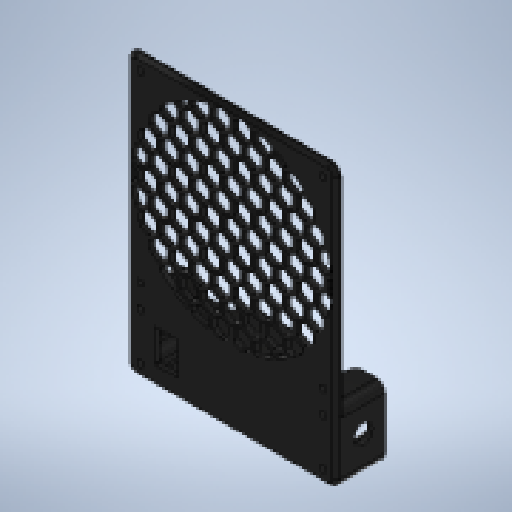
# Autodesk Inventor part: Face Plate
Saved by Autodesk Inventor 2023.2 (Build 272271000, 271)
## iProperties
Created: 2023-08-15
Part Number: Face Plate
Material: UHMW, Black
Document SubType Name: Modeling
Designer: Nathan Cai
Density: 0.94 g/cm^3
Appearance: Smooth - Black
Author: Nathan Cai
Autodesk Inventor part; units mm, degrees
ref_plane "YZ Plane" through (0, 0, 0) normal (1, 0, 0) x (0, 1, 0)
ref_plane "XZ Plane" through (0, 0, 0) normal (0, 1, 0) x (-1, 0, 0)
ref_plane "XY Plane" through (0, 0, 0) normal (0, 0, 1) x (1, 0, 0)
sketch "Sketch1" plane through (0, 0, 0) normal (0, 0, 1) x (1, 0, 0)
  line L0 (-60, -80) -> (60, -80)
  line L1 (60, -80) -> (60, 80)
  line L2 (60, 80) -> (-60, 80)
  line L3 (-60, 80) -> (-60, -80)
  line L4 (-60, -80) -> (60, 80) construction
  line L5 (60, -80) -> (-60, 80) construction
  line L6 (0, 80) -> (0, -80) construction
  line L7 (-52.5, 72.5) -> (52.5, 72.5) construction
  line L8 (52.5, 72.5) -> (52.5, -32.5) construction
  line L9 (52.5, -32.5) -> (-52.5, -32.5) construction
  line L10 (-52.5, -32.5) -> (-52.5, 72.5) construction
  line L11 (-52.5, 72.5) -> (52.5, -32.5) construction
  line L12 (52.5, 72.5) -> (-52.5, -32.5) construction
  circle A0 centre (-52.5, 72.5) radius 2
  circle A1 centre (52.5, 72.5) radius 2
  circle A2 centre (-52.5, -32.5) radius 2
  circle A3 centre (52.5, -32.5) radius 2
  circle A4 centre (-52.5, -72.5) radius 2
  circle A5 centre (52.5, -72.5) radius 2
  circle A6 centre (0, 20) radius 57.5
  circle A7 centre (52.5, -45.5) radius 2
  circle A8 centre (-52.5, -45.5) radius 2
  point P0 (0, 0)
  point P1 (0, 20)
  dimension "d0" = 120
  dimension "d1" = 160
  dimension "d2" = 105
  dimension "d3" = 105
  dimension "d4" = 7.5
  dimension "d5" = 4
  dimension "d8" = 105
  dimension "d11" = 105
  dimension "d16" = 40
  dimension "d21" = 115
  dimension "d82" = 13
  constraints: 26 end point, 9 centre point, 6 midpoint, 4 parallel, 3 horizontal, 3 vertical, 2 coincident, 2 perpendicular, 1 point on line, 14 other
  measures "d0" distance of L2.end L1.end
  measures "d1" distance of L1.end L0.end
  measures "d2" distance of L8.end L9.end
  measures "d3" distance of L7.end L8.end
  measures "d4" distance between parallel lines of L2 L7
  measures "d5" diameter of A0
  measures "d8" distance of A0.centre A1.centre
  measures "d11" distance of A0.centre A2.centre
  measures "d16" distance of A2.centre A4.centre
  measures "d21" diameter of A6
  measures "d82" distance of A3.centre A7.centre
extrude "Extrusion1" add sketch "Sketch1" along normal blind 3
sketch "Sketch2" plane through (0, 0, 3) normal (0, 0, 1) x (1, 0, 0)
  line L0 (60, -80) -> (60, 80) projected
  line L1 (60, 80) -> (-60, 80) projected
  line L2 (-60, 80) -> (-60, -80) projected
  line L3 (-60, -80) -> (60, -80) projected
  circle A0 centre (-52.5, -72.5) radius 2 projected
  circle A1 centre (52.5, -72.5) radius 2 projected
  circle A2 centre (0, 20) radius 57.5 projected
  circle A3 centre (52.5, -32.5) radius 2 projected
  circle A4 centre (-52.5, -32.5) radius 2 projected
  circle A5 centre (52.5, 72.5) radius 2 projected
  circle A6 centre (-52.5, 72.5) radius 2 projected
  circle A7 centre (0, 20) radius 18
  circle A8 centre (0, 20) radius 57.5 projected
  line L4 (0, 77.5) -> (0, -37.5) construction
  line L5 (0, 20) -> (-57.5, 20) construction
  line L6 (0, 25.7735) -> (5, 22.8868)
  line L7 (5, 22.8868) -> (5, 17.1132)
  line L8 (5, 17.1132) -> (0, 14.2265)
  line L9 (0, 14.2265) -> (-5, 17.1132)
  line L10 (-5, 17.1132) -> (-5, 22.8868)
  line L11 (-5, 22.8868) -> (0, 25.7735)
  line L12 (-17, 22.8868) -> (-12, 25.7735)
  line L13 (-7, 17.1132) -> (-12, 14.2265)
  line L14 (-12, 14.2265) -> (-17, 17.1132)
  line L15 (-17, 17.1132) -> (-17, 22.8868)
  line L16 (-7, 22.8868) -> (-7, 17.1132)
  line L17 (-12, 25.7735) -> (-7, 22.8868)
  line L18 (-29, 22.8868) -> (-24, 25.7735)
  line L19 (-19, 17.1132) -> (-24, 14.2265)
  line L20 (-24, 14.2265) -> (-29, 17.1132)
  line L21 (-29, 17.1132) -> (-29, 22.8868)
  line L22 (-19, 22.8868) -> (-19, 17.1132)
  line L23 (-24, 25.7735) -> (-19, 22.8868)
  line L24 (-41, 22.8868) -> (-36, 25.7735)
  line L25 (-31, 17.1132) -> (-36, 14.2265)
  line L26 (-36, 14.2265) -> (-41, 17.1132)
  line L27 (-41, 17.1132) -> (-41, 22.8868)
  line L28 (-31, 22.8868) -> (-31, 17.1132)
  line L29 (-36, 25.7735) -> (-31, 22.8868)
  line L30 (-53, 22.8868) -> (-48, 25.7735)
  line L31 (-43, 17.1132) -> (-48, 14.2265)
  line L32 (-48, 14.2265) -> (-53, 17.1132)
  line L33 (-53, 17.1132) -> (-53, 22.8868)
  line L34 (-43, 22.8868) -> (-43, 17.1132)
  line L35 (-48, 25.7735) -> (-43, 22.8868)
  line L36 (-65, 22.8868) -> (-60, 25.7735)
  line L37 (-55, 17.1132) -> (-60, 14.2265)
  line L38 (-60, 14.2265) -> (-65, 17.1132)
  line L39 (-65, 17.1132) -> (-65, 22.8868)
  line L40 (-55, 22.8868) -> (-55, 17.1132)
  line L41 (-60, 25.7735) -> (-55, 22.8868)
  line L42 (-6, 24.6188) -> (-11, 27.5056)
  line L43 (-11, 27.5056) -> (-11, 33.2791)
  line L44 (-11, 33.2791) -> (-6, 36.1658)
  line L45 (-6, 36.1658) -> (-1, 33.2791)
  line L46 (-1, 33.2791) -> (-1, 27.5056)
  line L47 (-1, 27.5056) -> (-6, 24.6188)
  line L48 (-18, 36.1658) -> (-13, 33.2791)
  line L49 (-13, 33.2791) -> (-13, 27.5056)
  line L50 (-13, 27.5056) -> (-18, 24.6188)
  line L51 (-23, 33.2791) -> (-18, 36.1658)
  line L52 (-23, 27.5056) -> (-23, 33.2791)
  line L53 (-18, 24.6188) -> (-23, 27.5056)
  line L54 (-30, 36.1658) -> (-25, 33.2791)
  line L55 (-25, 33.2791) -> (-25, 27.5056)
  line L56 (-25, 27.5056) -> (-30, 24.6188)
  line L57 (-35, 33.2791) -> (-30, 36.1658)
  line L58 (-35, 27.5056) -> (-35, 33.2791)
  line L59 (-30, 24.6188) -> (-35, 27.5056)
  line L60 (-42, 36.1658) -> (-37, 33.2791)
  line L61 (-37, 33.2791) -> (-37, 27.5056)
  line L62 (-37, 27.5056) -> (-42, 24.6188)
  line L63 (-47, 33.2791) -> (-42, 36.1658)
  line L64 (-47, 27.5056) -> (-47, 33.2791)
  line L65 (-42, 24.6188) -> (-47, 27.5056)
  line L66 (-54, 36.1658) -> (-49, 33.2791)
  line L67 (-49, 33.2791) -> (-49, 27.5056)
  line L68 (-49, 27.5056) -> (-54, 24.6188)
  line L69 (-59, 33.2791) -> (-54, 36.1658)
  line L70 (-59, 27.5056) -> (-59, 33.2791)
  line L71 (-54, 24.6188) -> (-59, 27.5056)
  line L72 (5, 43.6714) -> (5, 37.8979)
  line L73 (-5, 43.6714) -> (0, 46.5581)
  line L74 (-1, 48.2902) -> (-6, 45.4034)
  line L75 (-7, 43.6714) -> (-7, 37.8979)
  line L76 (0, 46.5581) -> (5, 43.6714)
  line L77 (-5, 37.8979) -> (-5, 43.6714)
  line L78 (-12, 46.5581) -> (-7, 43.6714)
  line L79 (-6, 45.4034) -> (-11, 48.2902)
  line L80 (5, 37.8979) -> (0, 35.0111)
  line L81 (0, 35.0111) -> (-5, 37.8979)
  line L82 (-7, 37.8979) -> (-12, 35.0111)
  line L83 (-11, 48.2902) -> (-11, 54.0637)
  line L84 (-1, 54.0637) -> (-1, 48.2902)
  line L85 (-11, 54.0637) -> (-6, 56.9504)
  line L86 (-6, 56.9504) -> (-1, 54.0637)
  line L87 (-24, 35.0111) -> (-29, 37.8979)
  line L88 (-29, 37.8979) -> (-29, 43.6714)
  line L89 (-31, 43.6714) -> (-31, 37.8979)
  line L90 (-31, 37.8979) -> (-36, 35.0111)
  line L91 (-41, 37.8979) -> (-41, 43.6714)
  line L92 (-36, 35.0111) -> (-41, 37.8979)
  line L93 (-53, 37.8979) -> (-53, 43.6714)
  line L94 (-48, 35.0111) -> (-53, 37.8979)
  line L95 (-43, 37.8979) -> (-48, 35.0111)
  line L96 (-43, 43.6714) -> (-43, 37.8979)
  line L97 (-65, 43.6714) -> (-60, 46.5581)
  line L98 (-60, 46.5581) -> (-55, 43.6714)
  line L99 (-55, 43.6714) -> (-55, 37.8979)
  line L100 (-55, 37.8979) -> (-60, 35.0111)
  line L101 (-65, 37.8979) -> (-65, 43.6714)
  line L102 (-60, 35.0111) -> (-65, 37.8979)
  line L103 (-17, 43.6714) -> (-12, 46.5581)
  line L104 (-12, 35.0111) -> (-17, 37.8979)
  line L105 (-17, 37.8979) -> (-17, 43.6714)
  line L106 (-19, 37.8979) -> (-24, 35.0111)
  line L107 (-13, 54.0637) -> (-13, 48.2902)
  line L108 (-18, 56.9504) -> (-13, 54.0637)
  line L109 (-13, 48.2902) -> (-18, 45.4034)
  line L110 (-23, 54.0637) -> (-18, 56.9504)
  line L111 (-23, 48.2902) -> (-23, 54.0637)
  line L112 (-18, 45.4034) -> (-23, 48.2902)
  line L113 (-19, 43.6714) -> (-19, 37.8979)
  line L114 (-24, 46.5581) -> (-19, 43.6714)
  line L115 (-29, 43.6714) -> (-24, 46.5581)
  line L116 (-36, 46.5581) -> (-31, 43.6714)
  line L117 (-41, 43.6714) -> (-36, 46.5581)
  line L118 (-30, 45.4034) -> (-35, 48.2902)
  line L119 (-37, 48.2902) -> (-42, 45.4034)
  line L120 (-25, 48.2902) -> (-30, 45.4034)
  line L121 (-42, 56.9504) -> (-37, 54.0637)
  line L122 (-37, 54.0637) -> (-37, 48.2902)
  line L123 (-35, 54.0637) -> (-30, 56.9504)
  line L124 (-25, 54.0637) -> (-25, 48.2902)
  line L125 (-30, 56.9504) -> (-25, 54.0637)
  line L126 (-35, 48.2902) -> (-35, 54.0637)
  line L127 (-53, 43.6714) -> (-48, 46.5581)
  line L128 (-48, 46.5581) -> (-43, 43.6714)
  line L129 (-42, 45.4034) -> (-47, 48.2902)
  line L130 (-49, 48.2902) -> (-54, 45.4034)
  line L131 (-54, 45.4034) -> (-59, 48.2902)
  line L132 (-47, 54.0637) -> (-42, 56.9504)
  line L133 (-49, 54.0637) -> (-49, 48.2902)
  line L134 (-54, 56.9504) -> (-49, 54.0637)
  line L135 (-59, 48.2902) -> (-59, 54.0637)
  line L136 (-59, 54.0637) -> (-54, 56.9504)
  line L137 (-47, 48.2902) -> (-47, 54.0637)
  line L138 (5, 64.456) -> (5, 58.6825)
  line L139 (-5, 64.456) -> (0, 67.3427)
  line L140 (-1, 69.0748) -> (-6, 66.188)
  line L141 (-7, 64.456) -> (-7, 58.6825)
  line L142 (0, 67.3427) -> (5, 64.456)
  line L143 (-5, 58.6825) -> (-5, 64.456)
  line L144 (-12, 67.3427) -> (-7, 64.456)
  line L145 (-6, 66.188) -> (-11, 69.0748)
  line L146 (5, 58.6825) -> (0, 55.7957)
  line L147 (0, 55.7957) -> (-5, 58.6825)
  line L148 (-7, 58.6825) -> (-12, 55.7957)
  line L149 (-11, 69.0748) -> (-11, 74.8483)
  line L150 (-1, 74.8483) -> (-1, 69.0748)
  line L151 (-11, 74.8483) -> (-6, 77.735)
  line L152 (-6, 77.735) -> (-1, 74.8483)
  line L153 (-24, 55.7957) -> (-29, 58.6825)
  line L154 (-29, 58.6825) -> (-29, 64.456)
  line L155 (-31, 64.456) -> (-31, 58.6825)
  line L156 (-31, 58.6825) -> (-36, 55.7957)
  line L157 (-41, 58.6825) -> (-41, 64.456)
  line L158 (-36, 55.7957) -> (-41, 58.6825)
  line L159 (-53, 58.6825) -> (-53, 64.456)
  line L160 (-48, 55.7957) -> (-53, 58.6825)
  line L161 (-43, 58.6825) -> (-48, 55.7957)
  line L162 (-43, 64.456) -> (-43, 58.6825)
  line L163 (-65, 64.456) -> (-60, 67.3427)
  line L164 (-60, 67.3427) -> (-55, 64.456)
  line L165 (-55, 64.456) -> (-55, 58.6825)
  line L166 (-55, 58.6825) -> (-60, 55.7957)
  line L167 (-65, 58.6825) -> (-65, 64.456)
  line L168 (-60, 55.7957) -> (-65, 58.6825)
  line L169 (-17, 64.456) -> (-12, 67.3427)
  line L170 (-12, 55.7957) -> (-17, 58.6825)
  line L171 (-17, 58.6825) -> (-17, 64.456)
  line L172 (-19, 58.6825) -> (-24, 55.7957)
  line L173 (-13, 74.8483) -> (-13, 69.0748)
  line L174 (-18, 77.735) -> (-13, 74.8483)
  line L175 (-13, 69.0748) -> (-18, 66.188)
  line L176 (-23, 74.8483) -> (-18, 77.735)
  line L177 (-23, 69.0748) -> (-23, 74.8483)
  line L178 (-18, 66.188) -> (-23, 69.0748)
  line L179 (-19, 64.456) -> (-19, 58.6825)
  line L180 (-24, 67.3427) -> (-19, 64.456)
  line L181 (-29, 64.456) -> (-24, 67.3427)
  line L182 (-36, 67.3427) -> (-31, 64.456)
  line L183 (-41, 64.456) -> (-36, 67.3427)
  line L184 (-30, 66.188) -> (-35, 69.0748)
  line L185 (-37, 69.0748) -> (-42, 66.188)
  line L186 (-25, 69.0748) -> (-30, 66.188)
  line L187 (-42, 77.735) -> (-37, 74.8483)
  line L188 (-37, 74.8483) -> (-37, 69.0748)
  line L189 (-35, 74.8483) -> (-30, 77.735)
  line L190 (-25, 74.8483) -> (-25, 69.0748)
  line L191 (-30, 77.735) -> (-25, 74.8483)
  line L192 (-35, 69.0748) -> (-35, 74.8483)
  line L193 (-53, 64.456) -> (-48, 67.3427)
  line L194 (-48, 67.3427) -> (-43, 64.456)
  line L195 (-42, 66.188) -> (-47, 69.0748)
  line L196 (-49, 69.0748) -> (-54, 66.188)
  line L197 (-54, 66.188) -> (-59, 69.0748)
  line L198 (-47, 74.8483) -> (-42, 77.735)
  line L199 (-49, 74.8483) -> (-49, 69.0748)
  line L200 (-54, 77.735) -> (-49, 74.8483)
  line L201 (-59, 69.0748) -> (-59, 74.8483)
  line L202 (-59, 74.8483) -> (-54, 77.735)
  line L203 (-47, 69.0748) -> (-47, 74.8483)
  line L204 (17, 22.8868) -> (12, 25.7735)
  line L205 (7, 17.1132) -> (12, 14.2265)
  line L206 (12, 14.2265) -> (17, 17.1132)
  line L207 (17, 17.1132) -> (17, 22.8868)
  line L208 (7, 22.8868) -> (7, 17.1132)
  line L209 (12, 25.7735) -> (7, 22.8868)
  line L210 (29, 22.8868) -> (24, 25.7735)
  line L211 (19, 17.1132) -> (24, 14.2265)
  line L212 (24, 14.2265) -> (29, 17.1132)
  line L213 (29, 17.1132) -> (29, 22.8868)
  line L214 (19, 22.8868) -> (19, 17.1132)
  line L215 (24, 25.7735) -> (19, 22.8868)
  line L216 (41, 22.8868) -> (36, 25.7735)
  line L217 (31, 17.1132) -> (36, 14.2265)
  line L218 (36, 14.2265) -> (41, 17.1132)
  line L219 (41, 17.1132) -> (41, 22.8868)
  line L220 (31, 22.8868) -> (31, 17.1132)
  line L221 (36, 25.7735) -> (31, 22.8868)
  line L222 (53, 22.8868) -> (48, 25.7735)
  line L223 (43, 17.1132) -> (48, 14.2265)
  line L224 (48, 14.2265) -> (53, 17.1132)
  line L225 (53, 17.1132) -> (53, 22.8868)
  line L226 (43, 22.8868) -> (43, 17.1132)
  line L227 (48, 25.7735) -> (43, 22.8868)
  line L228 (65, 22.8868) -> (60, 25.7735)
  line L229 (55, 17.1132) -> (60, 14.2265)
  line L230 (60, 14.2265) -> (65, 17.1132)
  line L231 (65, 17.1132) -> (65, 22.8868)
  line L232 (55, 22.8868) -> (55, 17.1132)
  line L233 (60, 25.7735) -> (55, 22.8868)
  line L234 (6, 24.6188) -> (11, 27.5056)
  line L235 (11, 27.5056) -> (11, 33.2791)
  line L236 (11, 33.2791) -> (6, 36.1658)
  line L237 (6, 36.1658) -> (1, 33.2791)
  line L238 (1, 33.2791) -> (1, 27.5056)
  line L239 (1, 27.5056) -> (6, 24.6188)
  line L240 (18, 36.1658) -> (13, 33.2791)
  line L241 (13, 33.2791) -> (13, 27.5056)
  line L242 (13, 27.5056) -> (18, 24.6188)
  line L243 (23, 33.2791) -> (18, 36.1658)
  line L244 (23, 27.5056) -> (23, 33.2791)
  line L245 (18, 24.6188) -> (23, 27.5056)
  line L246 (30, 36.1658) -> (25, 33.2791)
  line L247 (25, 33.2791) -> (25, 27.5056)
  line L248 (25, 27.5056) -> (30, 24.6188)
  line L249 (35, 33.2791) -> (30, 36.1658)
  line L250 (35, 27.5056) -> (35, 33.2791)
  line L251 (30, 24.6188) -> (35, 27.5056)
  line L252 (42, 36.1658) -> (37, 33.2791)
  line L253 (37, 33.2791) -> (37, 27.5056)
  line L254 (37, 27.5056) -> (42, 24.6188)
  line L255 (47, 33.2791) -> (42, 36.1658)
  line L256 (47, 27.5056) -> (47, 33.2791)
  line L257 (42, 24.6188) -> (47, 27.5056)
  line L258 (54, 36.1658) -> (49, 33.2791)
  line L259 (49, 33.2791) -> (49, 27.5056)
  line L260 (49, 27.5056) -> (54, 24.6188)
  line L261 (59, 33.2791) -> (54, 36.1658)
  line L262 (59, 27.5056) -> (59, 33.2791)
  line L263 (54, 24.6188) -> (59, 27.5056)
  line L264 (1, 48.2902) -> (6, 45.4034)
  line L265 (7, 43.6714) -> (7, 37.8979)
  line L266 (12, 46.5581) -> (7, 43.6714)
  line L267 (6, 45.4034) -> (11, 48.2902)
  line L268 (7, 37.8979) -> (12, 35.0111)
  line L269 (11, 48.2902) -> (11, 54.0637)
  line L270 (1, 54.0637) -> (1, 48.2902)
  line L271 (11, 54.0637) -> (6, 56.9504)
  line L272 (6, 56.9504) -> (1, 54.0637)
  line L273 (24, 35.0111) -> (29, 37.8979)
  line L274 (29, 37.8979) -> (29, 43.6714)
  line L275 (31, 43.6714) -> (31, 37.8979)
  line L276 (31, 37.8979) -> (36, 35.0111)
  line L277 (41, 37.8979) -> (41, 43.6714)
  line L278 (36, 35.0111) -> (41, 37.8979)
  line L279 (53, 37.8979) -> (53, 43.6714)
  line L280 (48, 35.0111) -> (53, 37.8979)
  line L281 (43, 37.8979) -> (48, 35.0111)
  line L282 (43, 43.6714) -> (43, 37.8979)
  line L283 (65, 43.6714) -> (60, 46.5581)
  line L284 (60, 46.5581) -> (55, 43.6714)
  line L285 (55, 43.6714) -> (55, 37.8979)
  line L286 (55, 37.8979) -> (60, 35.0111)
  line L287 (65, 37.8979) -> (65, 43.6714)
  line L288 (60, 35.0111) -> (65, 37.8979)
  line L289 (17, 43.6714) -> (12, 46.5581)
  line L290 (12, 35.0111) -> (17, 37.8979)
  line L291 (17, 37.8979) -> (17, 43.6714)
  line L292 (19, 37.8979) -> (24, 35.0111)
  line L293 (13, 54.0637) -> (13, 48.2902)
  line L294 (18, 56.9504) -> (13, 54.0637)
  line L295 (13, 48.2902) -> (18, 45.4034)
  line L296 (23, 54.0637) -> (18, 56.9504)
  line L297 (23, 48.2902) -> (23, 54.0637)
  line L298 (18, 45.4034) -> (23, 48.2902)
  line L299 (19, 43.6714) -> (19, 37.8979)
  line L300 (24, 46.5581) -> (19, 43.6714)
  line L301 (29, 43.6714) -> (24, 46.5581)
  line L302 (36, 46.5581) -> (31, 43.6714)
  line L303 (41, 43.6714) -> (36, 46.5581)
  line L304 (30, 45.4034) -> (35, 48.2902)
  line L305 (37, 48.2902) -> (42, 45.4034)
  line L306 (25, 48.2902) -> (30, 45.4034)
  line L307 (42, 56.9504) -> (37, 54.0637)
  line L308 (37, 54.0637) -> (37, 48.2902)
  line L309 (35, 54.0637) -> (30, 56.9504)
  line L310 (25, 54.0637) -> (25, 48.2902)
  line L311 (30, 56.9504) -> (25, 54.0637)
  line L312 (35, 48.2902) -> (35, 54.0637)
  line L313 (53, 43.6714) -> (48, 46.5581)
  line L314 (48, 46.5581) -> (43, 43.6714)
  line L315 (42, 45.4034) -> (47, 48.2902)
  line L316 (49, 48.2902) -> (54, 45.4034)
  line L317 (54, 45.4034) -> (59, 48.2902)
  line L318 (47, 54.0637) -> (42, 56.9504)
  line L319 (49, 54.0637) -> (49, 48.2902)
  line L320 (54, 56.9504) -> (49, 54.0637)
  line L321 (59, 48.2902) -> (59, 54.0637)
  line L322 (59, 54.0637) -> (54, 56.9504)
  line L323 (47, 48.2902) -> (47, 54.0637)
  line L324 (1, 69.0748) -> (6, 66.188)
  line L325 (7, 64.456) -> (7, 58.6825)
  line L326 (12, 67.3427) -> (7, 64.456)
  line L327 (6, 66.188) -> (11, 69.0748)
  line L328 (7, 58.6825) -> (12, 55.7957)
  line L329 (11, 69.0748) -> (11, 74.8483)
  line L330 (1, 74.8483) -> (1, 69.0748)
  line L331 (11, 74.8483) -> (6, 77.735)
  line L332 (6, 77.735) -> (1, 74.8483)
  line L333 (24, 55.7957) -> (29, 58.6825)
  line L334 (29, 58.6825) -> (29, 64.456)
  line L335 (31, 64.456) -> (31, 58.6825)
  line L336 (31, 58.6825) -> (36, 55.7957)
  line L337 (41, 58.6825) -> (41, 64.456)
  line L338 (36, 55.7957) -> (41, 58.6825)
  line L339 (53, 58.6825) -> (53, 64.456)
  line L340 (48, 55.7957) -> (53, 58.6825)
  line L341 (43, 58.6825) -> (48, 55.7957)
  line L342 (43, 64.456) -> (43, 58.6825)
  line L343 (65, 64.456) -> (60, 67.3427)
  line L344 (60, 67.3427) -> (55, 64.456)
  line L345 (55, 64.456) -> (55, 58.6825)
  line L346 (55, 58.6825) -> (60, 55.7957)
  line L347 (65, 58.6825) -> (65, 64.456)
  line L348 (60, 55.7957) -> (65, 58.6825)
  line L349 (17, 64.456) -> (12, 67.3427)
  line L350 (12, 55.7957) -> (17, 58.6825)
  line L351 (17, 58.6825) -> (17, 64.456)
  line L352 (19, 58.6825) -> (24, 55.7957)
  line L353 (13, 74.8483) -> (13, 69.0748)
  line L354 (18, 77.735) -> (13, 74.8483)
  line L355 (13, 69.0748) -> (18, 66.188)
  line L356 (23, 74.8483) -> (18, 77.735)
  line L357 (23, 69.0748) -> (23, 74.8483)
  line L358 (18, 66.188) -> (23, 69.0748)
  line L359 (19, 64.456) -> (19, 58.6825)
  line L360 (24, 67.3427) -> (19, 64.456)
  line L361 (29, 64.456) -> (24, 67.3427)
  line L362 (36, 67.3427) -> (31, 64.456)
  line L363 (41, 64.456) -> (36, 67.3427)
  line L364 (30, 66.188) -> (35, 69.0748)
  line L365 (37, 69.0748) -> (42, 66.188)
  line L366 (25, 69.0748) -> (30, 66.188)
  line L367 (42, 77.735) -> (37, 74.8483)
  line L368 (37, 74.8483) -> (37, 69.0748)
  line L369 (35, 74.8483) -> (30, 77.735)
  line L370 (25, 74.8483) -> (25, 69.0748)
  line L371 (30, 77.735) -> (25, 74.8483)
  line L372 (35, 69.0748) -> (35, 74.8483)
  line L373 (53, 64.456) -> (48, 67.3427)
  line L374 (48, 67.3427) -> (43, 64.456)
  line L375 (42, 66.188) -> (47, 69.0748)
  line L376 (49, 69.0748) -> (54, 66.188)
  line L377 (54, 66.188) -> (59, 69.0748)
  line L378 (47, 74.8483) -> (42, 77.735)
  line L379 (49, 74.8483) -> (49, 69.0748)
  line L380 (54, 77.735) -> (49, 74.8483)
  line L381 (59, 69.0748) -> (59, 74.8483)
  line L382 (59, 74.8483) -> (54, 77.735)
  line L383 (47, 69.0748) -> (47, 74.8483)
  line L384 (60, -40) -> (-60, -40)
  circle A9 centre (52.5, -32.5) radius 2
  circle A10 centre (-52.5, -32.5) radius 2
  line L385 (-6, 15.3812) -> (-11, 12.4944)
  line L386 (-11, 12.4944) -> (-11, 6.7209)
  line L387 (-11, 6.7209) -> (-6, 3.8342)
  line L388 (-6, 3.8342) -> (-1, 6.7209)
  line L389 (-1, 6.7209) -> (-1, 12.4944)
  line L390 (-1, 12.4944) -> (-6, 15.3812)
  line L391 (-18, 3.8342) -> (-13, 6.7209)
  line L392 (-13, 6.7209) -> (-13, 12.4944)
  line L393 (-13, 12.4944) -> (-18, 15.3812)
  line L394 (-23, 6.7209) -> (-18, 3.8342)
  line L395 (-23, 12.4944) -> (-23, 6.7209)
  line L396 (-18, 15.3812) -> (-23, 12.4944)
  line L397 (-30, 3.8342) -> (-25, 6.7209)
  line L398 (-25, 6.7209) -> (-25, 12.4944)
  line L399 (-25, 12.4944) -> (-30, 15.3812)
  line L400 (-35, 6.7209) -> (-30, 3.8342)
  line L401 (-35, 12.4944) -> (-35, 6.7209)
  line L402 (-30, 15.3812) -> (-35, 12.4944)
  line L403 (-42, 3.8342) -> (-37, 6.7209)
  line L404 (-37, 6.7209) -> (-37, 12.4944)
  line L405 (-37, 12.4944) -> (-42, 15.3812)
  line L406 (-47, 6.7209) -> (-42, 3.8342)
  line L407 (-47, 12.4944) -> (-47, 6.7209)
  line L408 (-42, 15.3812) -> (-47, 12.4944)
  line L409 (-54, 3.8342) -> (-49, 6.7209)
  line L410 (-49, 6.7209) -> (-49, 12.4944)
  line L411 (-49, 12.4944) -> (-54, 15.3812)
  line L412 (-59, 6.7209) -> (-54, 3.8342)
  line L413 (-59, 12.4944) -> (-59, 6.7209)
  line L414 (-54, 15.3812) -> (-59, 12.4944)
  line L415 (5, -3.6714) -> (5, 2.1021)
  line L416 (-5, -3.6714) -> (0, -6.5581)
  line L417 (-1, -8.2902) -> (-6, -5.4034)
  line L418 (-7, -3.6714) -> (-7, 2.1021)
  line L419 (0, -6.5581) -> (5, -3.6714)
  line L420 (-5, 2.1021) -> (-5, -3.6714)
  line L421 (-12, -6.5581) -> (-7, -3.6714)
  line L422 (-6, -5.4034) -> (-11, -8.2902)
  line L423 (5, 2.1021) -> (0, 4.9889)
  line L424 (0, 4.9889) -> (-5, 2.1021)
  line L425 (-7, 2.1021) -> (-12, 4.9889)
  line L426 (-11, -8.2902) -> (-11, -14.0637)
  line L427 (-1, -14.0637) -> (-1, -8.2902)
  line L428 (-11, -14.0637) -> (-6, -16.9504)
  line L429 (-6, -16.9504) -> (-1, -14.0637)
  line L430 (-24, 4.9889) -> (-29, 2.1021)
  line L431 (-29, 2.1021) -> (-29, -3.6714)
  line L432 (-31, -3.6714) -> (-31, 2.1021)
  line L433 (-31, 2.1021) -> (-36, 4.9889)
  line L434 (-41, 2.1021) -> (-41, -3.6714)
  line L435 (-36, 4.9889) -> (-41, 2.1021)
  line L436 (-53, 2.1021) -> (-53, -3.6714)
  line L437 (-48, 4.9889) -> (-53, 2.1021)
  line L438 (-43, 2.1021) -> (-48, 4.9889)
  line L439 (-43, -3.6714) -> (-43, 2.1021)
  line L440 (-65, -3.6714) -> (-60, -6.5581)
  line L441 (-60, -6.5581) -> (-55, -3.6714)
  line L442 (-55, -3.6714) -> (-55, 2.1021)
  line L443 (-55, 2.1021) -> (-60, 4.9889)
  line L444 (-65, 2.1021) -> (-65, -3.6714)
  line L445 (-60, 4.9889) -> (-65, 2.1021)
  line L446 (-17, -3.6714) -> (-12, -6.5581)
  line L447 (-12, 4.9889) -> (-17, 2.1021)
  line L448 (-17, 2.1021) -> (-17, -3.6714)
  line L449 (-19, 2.1021) -> (-24, 4.9889)
  line L450 (-13, -14.0637) -> (-13, -8.2902)
  line L451 (-18, -16.9504) -> (-13, -14.0637)
  line L452 (-13, -8.2902) -> (-18, -5.4034)
  line L453 (-23, -14.0637) -> (-18, -16.9504)
  line L454 (-23, -8.2902) -> (-23, -14.0637)
  line L455 (-18, -5.4034) -> (-23, -8.2902)
  line L456 (-19, -3.6714) -> (-19, 2.1021)
  line L457 (-24, -6.5581) -> (-19, -3.6714)
  line L458 (-29, -3.6714) -> (-24, -6.5581)
  line L459 (-36, -6.5581) -> (-31, -3.6714)
  line L460 (-41, -3.6714) -> (-36, -6.5581)
  line L461 (-30, -5.4034) -> (-35, -8.2902)
  line L462 (-37, -8.2902) -> (-42, -5.4034)
  line L463 (-25, -8.2902) -> (-30, -5.4034)
  line L464 (-42, -16.9504) -> (-37, -14.0637)
  line L465 (-37, -14.0637) -> (-37, -8.2902)
  line L466 (-35, -14.0637) -> (-30, -16.9504)
  line L467 (-25, -14.0637) -> (-25, -8.2902)
  line L468 (-30, -16.9504) -> (-25, -14.0637)
  line L469 (-35, -8.2902) -> (-35, -14.0637)
  line L470 (-53, -3.6714) -> (-48, -6.5581)
  line L471 (-48, -6.5581) -> (-43, -3.6714)
  line L472 (-42, -5.4034) -> (-47, -8.2902)
  line L473 (-49, -8.2902) -> (-54, -5.4034)
  line L474 (-54, -5.4034) -> (-59, -8.2902)
  line L475 (-47, -14.0637) -> (-42, -16.9504)
  line L476 (-49, -14.0637) -> (-49, -8.2902)
  line L477 (-54, -16.9504) -> (-49, -14.0637)
  line L478 (-59, -8.2902) -> (-59, -14.0637)
  line L479 (-59, -14.0637) -> (-54, -16.9504)
  line L480 (-47, -8.2902) -> (-47, -14.0637)
  line L481 (5, -24.456) -> (5, -18.6825)
  line L482 (-5, -24.456) -> (0, -27.3427)
  line L483 (-1, -29.0748) -> (-6, -26.188)
  line L484 (-7, -24.456) -> (-7, -18.6825)
  line L485 (0, -27.3427) -> (5, -24.456)
  line L486 (-5, -18.6825) -> (-5, -24.456)
  line L487 (-12, -27.3427) -> (-7, -24.456)
  line L488 (-6, -26.188) -> (-11, -29.0748)
  line L489 (5, -18.6825) -> (0, -15.7957)
  line L490 (0, -15.7957) -> (-5, -18.6825)
  line L491 (-7, -18.6825) -> (-12, -15.7957)
  line L492 (-11, -29.0748) -> (-11, -34.8483)
  line L493 (-1, -34.8483) -> (-1, -29.0748)
  line L494 (-11, -34.8483) -> (-6, -37.735)
  line L495 (-6, -37.735) -> (-1, -34.8483)
  line L496 (-24, -15.7957) -> (-29, -18.6825)
  line L497 (-29, -18.6825) -> (-29, -24.456)
  line L498 (-31, -24.456) -> (-31, -18.6825)
  line L499 (-31, -18.6825) -> (-36, -15.7957)
  line L500 (-41, -18.6825) -> (-41, -24.456)
  line L501 (-36, -15.7957) -> (-41, -18.6825)
  line L502 (-53, -18.6825) -> (-53, -24.456)
  line L503 (-48, -15.7957) -> (-53, -18.6825)
  line L504 (-43, -18.6825) -> (-48, -15.7957)
  line L505 (-43, -24.456) -> (-43, -18.6825)
  line L506 (-65, -24.456) -> (-60, -27.3427)
  line L507 (-60, -27.3427) -> (-55, -24.456)
  line L508 (-55, -24.456) -> (-55, -18.6825)
  line L509 (-55, -18.6825) -> (-60, -15.7957)
  line L510 (-65, -18.6825) -> (-65, -24.456)
  line L511 (-60, -15.7957) -> (-65, -18.6825)
  line L512 (-17, -24.456) -> (-12, -27.3427)
  line L513 (-12, -15.7957) -> (-17, -18.6825)
  line L514 (-17, -18.6825) -> (-17, -24.456)
  line L515 (-19, -18.6825) -> (-24, -15.7957)
  line L516 (-13, -34.8483) -> (-13, -29.0748)
  line L517 (-18, -37.735) -> (-13, -34.8483)
  line L518 (-13, -29.0748) -> (-18, -26.188)
  line L519 (-23, -34.8483) -> (-18, -37.735)
  line L520 (-23, -29.0748) -> (-23, -34.8483)
  line L521 (-18, -26.188) -> (-23, -29.0748)
  line L522 (-19, -24.456) -> (-19, -18.6825)
  line L523 (-24, -27.3427) -> (-19, -24.456)
  line L524 (-29, -24.456) -> (-24, -27.3427)
  line L525 (-36, -27.3427) -> (-31, -24.456)
  line L526 (-41, -24.456) -> (-36, -27.3427)
  line L527 (-30, -26.188) -> (-35, -29.0748)
  line L528 (-37, -29.0748) -> (-42, -26.188)
  line L529 (-25, -29.0748) -> (-30, -26.188)
  line L530 (-42, -37.735) -> (-37, -34.8483)
  line L531 (-37, -34.8483) -> (-37, -29.0748)
  line L532 (-35, -34.8483) -> (-30, -37.735)
  line L533 (-25, -34.8483) -> (-25, -29.0748)
  line L534 (-30, -37.735) -> (-25, -34.8483)
  line L535 (-35, -29.0748) -> (-35, -34.8483)
  line L536 (-53, -24.456) -> (-48, -27.3427)
  line L537 (-48, -27.3427) -> (-43, -24.456)
  line L538 (-42, -26.188) -> (-47, -29.0748)
  line L539 (-49, -29.0748) -> (-54, -26.188)
  line L540 (-54, -26.188) -> (-59, -29.0748)
  line L541 (-47, -34.8483) -> (-42, -37.735)
  line L542 (-49, -34.8483) -> (-49, -29.0748)
  line L543 (-54, -37.735) -> (-49, -34.8483)
  line L544 (-59, -29.0748) -> (-59, -34.8483)
  line L545 (-59, -34.8483) -> (-54, -37.735)
  line L546 (-47, -29.0748) -> (-47, -34.8483)
  line L547 (6, 15.3812) -> (11, 12.4944)
  line L548 (11, -8.2902) -> (11, -14.0637)
  line L549 (11, -14.0637) -> (6, -16.9504)
  line L550 (7, -18.6825) -> (12, -15.7957)
  line L551 (12, -27.3427) -> (7, -24.456)
  line L552 (7, -24.456) -> (7, -18.6825)
  line L553 (11, 6.7209) -> (6, 3.8342)
  line L554 (7, -3.6714) -> (7, 2.1021)
  line L555 (7, 2.1021) -> (12, 4.9889)
  line L556 (12, 4.9889) -> (17, 2.1021)
  line L557 (17, 2.1021) -> (17, -3.6714)
  line L558 (6, -5.4034) -> (11, -8.2902)
  line L559 (17, -3.6714) -> (12, -6.5581)
  line L560 (13, -14.0637) -> (13, -8.2902)
  line L561 (13, -8.2902) -> (18, -5.4034)
  line L562 (12, -6.5581) -> (7, -3.6714)
  line L563 (6, -26.188) -> (11, -29.0748)
  line L564 (11, -29.0748) -> (11, -34.8483)
  line L565 (18, -37.735) -> (13, -34.8483)
  line L566 (13, -34.8483) -> (13, -29.0748)
  line L567 (11, -34.8483) -> (6, -37.735)
  line L568 (19, -3.6714) -> (19, 2.1021)
  line L569 (23, -8.2902) -> (23, -14.0637)
  line L570 (18, -5.4034) -> (23, -8.2902)
  line L571 (19, 2.1021) -> (24, 4.9889)
  line L572 (24, -6.5581) -> (19, -3.6714)
  line L573 (24, 4.9889) -> (29, 2.1021)
  line L574 (18, 15.3812) -> (23, 12.4944)
  line L575 (25, 6.7209) -> (25, 12.4944)
  line L576 (23, 12.4944) -> (23, 6.7209)
  line L577 (13, 12.4944) -> (18, 15.3812)
  line L578 (11, 12.4944) -> (11, 6.7209)
  line L579 (13, 6.7209) -> (13, 12.4944)
  line L580 (18, 3.8342) -> (13, 6.7209)
  line L581 (23, 6.7209) -> (18, 3.8342)
  line L582 (30, 3.8342) -> (25, 6.7209)
  line L583 (25, 12.4944) -> (30, 15.3812)
  line L584 (18, -16.9504) -> (13, -14.0637)
  line L585 (23, -14.0637) -> (18, -16.9504)
  line L586 (30, -16.9504) -> (25, -14.0637)
  line L587 (17, -24.456) -> (12, -27.3427)
  line L588 (12, -15.7957) -> (17, -18.6825)
  line L589 (13, -29.0748) -> (18, -26.188)
  line L590 (17, -18.6825) -> (17, -24.456)
  line L591 (19, -24.456) -> (19, -18.6825)
  line L592 (18, -26.188) -> (23, -29.0748)
  line L593 (24, -27.3427) -> (19, -24.456)
  line L594 (19, -18.6825) -> (24, -15.7957)
  line L595 (24, -15.7957) -> (29, -18.6825)
  line L596 (36, -6.5581) -> (31, -3.6714)
  line L597 (41, -3.6714) -> (36, -6.5581)
  line L598 (30, -5.4034) -> (35, -8.2902)
  line L599 (29, -3.6714) -> (24, -6.5581)
  line L600 (25, -8.2902) -> (30, -5.4034)
  line L601 (25, -14.0637) -> (25, -8.2902)
  line L602 (37, -8.2902) -> (42, -5.4034)
  line L603 (35, -8.2902) -> (35, -14.0637)
  line L604 (37, -14.0637) -> (37, -8.2902)
  line L605 (35, -14.0637) -> (30, -16.9504)
  line L606 (31, -18.6825) -> (36, -15.7957)
  line L607 (42, -16.9504) -> (37, -14.0637)
  line L608 (29, -18.6825) -> (29, -24.456)
  line L609 (31, -24.456) -> (31, -18.6825)
  line L610 (36, -15.7957) -> (41, -18.6825)
  line L611 (41, -18.6825) -> (41, -24.456)
  line L612 (23, -34.8483) -> (18, -37.735)
  line L613 (23, -29.0748) -> (23, -34.8483)
  line L614 (29, -24.456) -> (24, -27.3427)
  line L615 (25, -29.0748) -> (30, -26.188)
  line L616 (25, -34.8483) -> (25, -29.0748)
  line L617 (30, -26.188) -> (35, -29.0748)
  line L618 (36, -27.3427) -> (31, -24.456)
  line L619 (30, -37.735) -> (25, -34.8483)
  line L620 (35, -29.0748) -> (35, -34.8483)
  line L621 (35, -34.8483) -> (30, -37.735)
  line L622 (37, -34.8483) -> (37, -29.0748)
  line L623 (41, -24.456) -> (36, -27.3427)
  line L624 (37, -29.0748) -> (42, -26.188)
  line L625 (42, -37.735) -> (37, -34.8483)
  line L626 (29, 2.1021) -> (29, -3.6714)
  line L627 (41, 2.1021) -> (41, -3.6714)
  line L628 (43, -3.6714) -> (43, 2.1021)
  line L629 (43, 2.1021) -> (48, 4.9889)
  line L630 (36, 4.9889) -> (41, 2.1021)
  line L631 (31, -3.6714) -> (31, 2.1021)
  line L632 (31, 2.1021) -> (36, 4.9889)
  line L633 (42, 15.3812) -> (47, 12.4944)
  line L634 (37, 12.4944) -> (42, 15.3812)
  line L635 (47, 12.4944) -> (47, 6.7209)
  line L636 (47, 6.7209) -> (42, 3.8342)
  line L637 (37, 6.7209) -> (37, 12.4944)
  line L638 (42, 3.8342) -> (37, 6.7209)
  line L639 (35, 12.4944) -> (35, 6.7209)
  line L640 (35, 6.7209) -> (30, 3.8342)
  line L641 (30, 15.3812) -> (35, 12.4944)
  line L642 (53, -3.6714) -> (48, -6.5581)
  line L643 (48, -6.5581) -> (43, -3.6714)
  line L644 (42, -5.4034) -> (47, -8.2902)
  line L645 (49, -8.2902) -> (54, -5.4034)
  line L646 (47, -14.0637) -> (42, -16.9504)
  line L647 (43, -24.456) -> (43, -18.6825)
  line L648 (43, -18.6825) -> (48, -15.7957)
  line L649 (47, -8.2902) -> (47, -14.0637)
  line L650 (49, -14.0637) -> (49, -8.2902)
  line L651 (53, -18.6825) -> (53, -24.456)
  line L652 (48, -15.7957) -> (53, -18.6825)
  line L653 (54, -16.9504) -> (49, -14.0637)
  line L654 (54, 15.3812) -> (59, 12.4944)
  line L655 (49, 12.4944) -> (54, 15.3812)
  line L656 (59, 12.4944) -> (59, 6.7209)
  line L657 (49, 6.7209) -> (49, 12.4944)
  line L658 (59, 6.7209) -> (54, 3.8342)
  line L659 (55, 2.1021) -> (60, 4.9889)
  line L660 (54, 3.8342) -> (49, 6.7209)
  line L661 (48, 4.9889) -> (53, 2.1021)
  line L662 (53, -24.456) -> (48, -27.3427)
  line L663 (48, -27.3427) -> (43, -24.456)
  line L664 (49, -29.0748) -> (54, -26.188)
  line L665 (42, -26.188) -> (47, -29.0748)
  line L666 (60, -27.3427) -> (55, -24.456)
  line L667 (54, -26.188) -> (59, -29.0748)
  line L668 (47, -34.8483) -> (42, -37.735)
  line L669 (47, -29.0748) -> (47, -34.8483)
  line L670 (49, -34.8483) -> (49, -29.0748)
  line L671 (54, -37.735) -> (49, -34.8483)
  line L672 (59, -29.0748) -> (59, -34.8483)
  line L673 (59, -34.8483) -> (54, -37.735)
  line L674 (59, -14.0637) -> (54, -16.9504)
  line L675 (55, -18.6825) -> (60, -15.7957)
  line L676 (60, -15.7957) -> (65, -18.6825)
  line L677 (55, -24.456) -> (55, -18.6825)
  line L678 (65, -18.6825) -> (65, -24.456)
  line L679 (65, -24.456) -> (60, -27.3427)
  line L680 (60, 4.9889) -> (65, 2.1021)
  line L681 (53, 2.1021) -> (53, -3.6714)
  line L682 (55, -3.6714) -> (55, 2.1021)
  line L683 (65, 2.1021) -> (65, -3.6714)
  line L684 (60, -6.5581) -> (55, -3.6714)
  line L685 (54, -5.4034) -> (59, -8.2902)
  line L686 (65, -3.6714) -> (60, -6.5581)
  line L687 (59, -8.2902) -> (59, -14.0637)
  line L688 (6, 3.8342) -> (1, 6.7209)
  line L689 (1, 6.7209) -> (1, 12.4944)
  line L690 (1, 12.4944) -> (6, 15.3812)
  line L691 (1, -8.2902) -> (6, -5.4034)
  line L692 (1, -14.0637) -> (1, -8.2902)
  line L693 (6, -16.9504) -> (1, -14.0637)
  line L694 (1, -29.0748) -> (6, -26.188)
  line L695 (1, -34.8483) -> (1, -29.0748)
  line L696 (6, -37.735) -> (1, -34.8483)
  point P0 (0, 0)
  point P1 (-12, 20)
  point P2 (-12, 20)
  point P3 (-12, 20)
  point P4 (-12, 20)
  point P5 (-24, 20)
  point P6 (-24, 20)
  point P7 (-24, 20)
  point P8 (-24, 20)
  point P9 (-36, 20)
  point P10 (-36, 20)
  point P11 (-36, 20)
  point P12 (-36, 20)
  point P13 (-48, 20)
  point P14 (-48, 20)
  point P15 (-48, 20)
  point P16 (-48, 20)
  point P17 (-60, 20)
  point P18 (-60, 20)
  point P19 (-60, 20)
  point P20 (-60, 20)
  point P21 (-6, 30.3923)
  point P22 (-18, 30.3923)
  point P23 (-30, 30.3923)
  point P24 (-42, 30.3923)
  point P25 (-54, 30.3923)
  point P26 (0, 40.7846)
  point P27 (0, 40.7846)
  point P28 (0, 40.7846)
  point P29 (0, 40.7846)
  point P30 (0, 40.7846)
  point P31 (-12, 40.7846)
  point P32 (-12, 40.7846)
  point P33 (-12, 40.7846)
  point P34 (-12, 40.7846)
  point P35 (-6, 51.1769)
  point P36 (-57.5, 40.7846)
  point P37 (-36, 40.7846)
  point P38 (-36, 40.7846)
  point P39 (-36, 40.7846)
  point P40 (-36, 40.7846)
  point P41 (-48, 40.7846)
  point P42 (-48, 40.7846)
  point P43 (-48, 40.7846)
  point P44 (-48, 40.7846)
  point P45 (-60, 40.7846)
  point P46 (-60, 40.7846)
  point P47 (-60, 40.7846)
  point P48 (-60, 40.7846)
  point P49 (-24, 40.7846)
  point P50 (-18, 51.1769)
  point P51 (-24, 40.7846)
  point P52 (-24, 40.7846)
  point P53 (-24, 40.7846)
  point P54 (-30, 51.1769)
  point P55 (-54, 51.1769)
  point P56 (-42, 51.1769)
  point P57 (0, 61.5692)
  point P58 (0, 61.5692)
  point P59 (0, 61.5692)
  point P60 (0, 61.5692)
  point P61 (0, 61.5692)
  point P62 (-12, 61.5692)
  point P63 (-12, 61.5692)
  point P64 (-12, 61.5692)
  point P65 (-12, 61.5692)
  point P66 (-6, 71.9615)
  point P67 (-57.5, 61.5692)
  point P68 (-36, 61.5692)
  point P69 (-36, 61.5692)
  point P70 (-36, 61.5692)
  point P71 (-36, 61.5692)
  point P72 (-48, 61.5692)
  point P73 (-48, 61.5692)
  point P74 (-48, 61.5692)
  point P75 (-48, 61.5692)
  point P76 (-60, 61.5692)
  point P77 (-60, 61.5692)
  point P78 (-60, 61.5692)
  point P79 (-60, 61.5692)
  point P80 (-24, 61.5692)
  point P81 (-18, 71.9615)
  point P82 (-24, 61.5692)
  point P83 (-24, 61.5692)
  point P84 (-24, 61.5692)
  point P85 (-30, 71.9615)
  point P86 (-54, 71.9615)
  point P87 (-42, 71.9615)
  point P88 (52.5, 72.5)
  point P89 (57.5, 20)
  point P90 (12, 20)
  point P91 (12, 20)
  point P92 (12, 20)
  point P93 (12, 20)
  point P94 (24, 20)
  point P95 (24, 20)
  point P96 (24, 20)
  point P97 (24, 20)
  point P98 (36, 20)
  point P99 (36, 20)
  point P100 (36, 20)
  point P101 (36, 20)
  point P102 (48, 20)
  point P103 (48, 20)
  point P104 (48, 20)
  point P105 (48, 20)
  point P106 (60, 20)
  point P107 (60, 20)
  point P108 (60, 20)
  point P109 (60, 20)
  point P110 (6, 30.3923)
  point P111 (18, 30.3923)
  point P112 (30, 30.3923)
  point P113 (42, 30.3923)
  point P114 (54, 30.3923)
  point P115 (12, 40.7846)
  point P116 (12, 40.7846)
  point P117 (12, 40.7846)
  point P118 (12, 40.7846)
  point P119 (6, 51.1769)
  point P120 (57.5, 40.7846)
  point P121 (36, 40.7846)
  point P122 (36, 40.7846)
  point P123 (36, 40.7846)
  point P124 (36, 40.7846)
  point P125 (48, 40.7846)
  point P126 (48, 40.7846)
  point P127 (48, 40.7846)
  point P128 (48, 40.7846)
  point P129 (60, 40.7846)
  point P130 (60, 40.7846)
  point P131 (60, 40.7846)
  point P132 (60, 40.7846)
  point P133 (24, 40.7846)
  point P134 (18, 51.1769)
  point P135 (24, 40.7846)
  point P136 (24, 40.7846)
  point P137 (24, 40.7846)
  point P138 (30, 51.1769)
  point P139 (54, 51.1769)
  point P140 (42, 51.1769)
  point P141 (12, 61.5692)
  point P142 (12, 61.5692)
  point P143 (12, 61.5692)
  point P144 (12, 61.5692)
  point P145 (6, 71.9615)
  point P146 (57.5, 61.5692)
  point P147 (36, 61.5692)
  point P148 (36, 61.5692)
  point P149 (36, 61.5692)
  point P150 (36, 61.5692)
  point P151 (48, 61.5692)
  point P152 (48, 61.5692)
  point P153 (48, 61.5692)
  point P154 (48, 61.5692)
  point P155 (60, 61.5692)
  point P156 (60, 61.5692)
  point P157 (60, 61.5692)
  point P158 (60, 61.5692)
  point P159 (24, 61.5692)
  point P160 (18, 71.9615)
  point P161 (24, 61.5692)
  point P162 (24, 61.5692)
  point P163 (24, 61.5692)
  point P164 (30, 71.9615)
  point P165 (54, 71.9615)
  point P166 (42, 71.9615)
  point P167 (-6, 9.6077)
  point P168 (-18, 9.6077)
  point P169 (-30, 9.6077)
  point P170 (-42, 9.6077)
  point P171 (-54, 9.6077)
  point P172 (0, -0.7846)
  point P173 (0, -0.7846)
  point P174 (0, -0.7846)
  point P175 (0, -0.7846)
  point P176 (0, -0.7846)
  point P177 (-12, -0.7846)
  point P178 (-12, -0.7846)
  point P179 (-12, -0.7846)
  point P180 (-12, -0.7846)
  point P181 (-6, -11.1769)
  point P182 (-57.5, -0.7846)
  point P183 (-36, -0.7846)
  point P184 (-36, -0.7846)
  point P185 (-36, -0.7846)
  point P186 (-36, -0.7846)
  point P187 (-48, -0.7846)
  point P188 (-48, -0.7846)
  point P189 (-48, -0.7846)
  point P190 (-48, -0.7846)
  point P191 (-60, -0.7846)
  point P192 (-60, -0.7846)
  point P193 (-60, -0.7846)
  point P194 (-60, -0.7846)
  point P195 (-24, -0.7846)
  point P196 (-18, -11.1769)
  point P197 (-24, -0.7846)
  point P198 (-24, -0.7846)
  point P199 (-24, -0.7846)
  dimension "d24" = 36
  dimension "d45" = 10
  dimension "d48" = 12
  dimension "d53" = 10
  dimension "d54" = 2
  dimension "d55" = 1
  dimension "d58" = 12
  dimension "d63" = 10.3923
  dimension "d66" = 20.7846
  constraints: 1386 end point, 700 symmetric about line, 110 coincident, 3 centre point, 3 horizontal, 3 point on circle, 2 midpoint, 2 vertical, 1 parallel, 1 point on line, 487 other
  measures "d24" diameter of A7
  measures "d45" distance between parallel lines of L7 L10
  measures "d48" distance of L6.start L12.end
  measures "d53" distance between parallel lines of L46 L43
  measures "d54" distance between parallel lines of L11 L47
  measures "d55" distance between parallel lines of L4 L46
  measures "d58" distance of L44.end L48.start
  measures "d63" vertical distance of point (0, 20) point (-6, 30.392)
  measures "d66" distance of L5.start point (0, 40.785)
extrude "Extrusion2" add sketch "Sketch2" against normal up to surface (3 mm away) contours A2 L654 L655 L657 L660 L658 L681 L661 L629 L628 L643 L642 L645 L650 L649 L644 L602 L604 L607 L646 L611 L610 L606 L609 L618 L617 L615 L616 L613 L592 L589 L566 L565 L567 L564 L563 L694 L695 L696 L495 L493 L483 L488 L492 L494 L517 L516 L518 L521 L520 L533 L529 L527 L525 L498 L499 L501 L500 L475 L464 L465 L462 L472 L480 L476 L473 L470 L471 L439 L438 L437 L436 L412 L409 L410 L411 L414 L37 L40 L41 L71 L68 L67 L66 L69 L93 L94 L95 L96 L128 L127 L130 L133 L137 L129 L119 L122 L121 L132 L157 L158 L156 L155 L182 L184 L186 L190 L177 L178 L175 L173 L174 L151 L149 L145 L140 L150 L152 L332 L330 L324 L327 L329 L331 L354 L353 L355 L358 L357 L370 L366 L364 L362 L335 L336 L338 L337 L318 L307 L308 L305 L315 L323 L319 L316 L313 L314 L282 L281 L280 L279 L261 L258 L259 L260 L263 L233 L232 L229 | A2 L650 L645 | L316 L319 A2 | L473 L476 A2 | A2 L133 L130 | A7 L577 L579 L423 L424 L392 L393 L50 L49 L81 L80 L241 L242
sketch "Sketch3" plane through (0, 0, 0) normal (0, 0, -1) x (-1, 0, 0)
  line L0 (-60, -80) -> (-60, 80) projected
  line L1 (-60, -80) -> (60, -80)
  line L2 (60, -80) -> (60, -40)
  line L3 (60, -40) -> (-60, -40)
  line L4 (-60, -40) -> (-60, -80)
  line L5 (-57, -43) -> (57, -43)
  line L6 (57, -43) -> (57, -77)
  line L7 (57, -77) -> (-57, -77)
  line L8 (-57, -77) -> (-57, -43)
  circle A0 centre (-52.5, -72.5) radius 2 projected
  circle A1 centre (-52.5, -72.5) radius 4.5
  line L9 (-48, -72.5) -> (-48, -77)
  line L10 (-52.5, -68) -> (-57, -68)
  line L11 (0, -77) -> (0, -43) construction
  circle A2 centre (52.5, -72.5) radius 2
  circle A3 centre (52.5, -72.5) radius 4.5
  line L12 (48, -72.5) -> (48, -77)
  line L13 (52.5, -68) -> (57, -68)
  line L14 (-60, 80) -> (60, 80) projected
  circle A4 centre (-52.5, -45.5) radius 2 projected
  arc A5 (-52.5, -50) -> (-48, -45.5) centre (-52.5, -45.5) ccw
  line L15 (-52.5, -50) -> (-57, -50)
  line L16 (-48, -45.5) -> (-48, -43)
  arc A6 (48, -45.5) -> (52.5, -50) centre (52.5, -45.5) ccw
  line L17 (52.5, -50) -> (57, -50)
  line L18 (48, -45.5) -> (48, -43)
  circle A7 centre (52.5, -45.5) radius 2 projected
  point P0 (0, 0)
  dimension "d74" = 120
  dimension "d75" = 40
  dimension "d76" = 3
  dimension "d77" = 160
  constraints: 34 end point, 11 symmetric about line, 8 point on circle, 6 perpendicular, 6 tangent, 5 centre point, 4 parallel, 4 point on line, 3 coincident, 2 midpoint, 1 horizontal, 6 other
  measures "d74" distance of L3.end L2.end
  measures "d75" distance of L2.end L1.end
  measures "d76" distance between parallel lines of L0 L8
  measures "d77" distance between parallel lines of L14 L1
extrude "Extrusion3" add sketch "Sketch3" along normal blind 25 contours L0 L3 L2 L1 | L5 L16 A5 L15 L8 | L5 L6 L17 A6 L18 | L10 A1 L8 | A1 L7 L8 | A1 | A1 L9 L7 | L6 A3 L13 | A3 | L6 L7 A3 | L12 A3 L7
sketch "Sketch6" plane through (0, 0, -25) normal (0, 0, -1) x (-1, 0, 0)
  line L0 (-48, -43) -> (48, -43) projected
  line L1 (60, -40) -> (-60, -40) projected
  line L2 (-43, -43) -> (-18, -43)
  line L3 (-18, -43) -> (-18, -40)
  line L4 (-18, -40) -> (-43, -40)
  line L5 (-43, -40) -> (-43, -43)
  line L6 (0, -40) -> (0, -43) construction
  line L7 (-48, -45.5) -> (-48, -43) projected
  line L8 (43, -43) -> (18, -43)
  line L9 (18, -43) -> (18, -40)
  line L10 (18, -40) -> (43, -40)
  line L11 (43, -40) -> (43, -43)
  point P0 (0, 0)
  point P1 (18, -40)
  point P2 (18, -43)
  dimension "d108" = 5
  dimension "d109" = 25
  constraints: 18 end point, 4 symmetric about line, 2 midpoint, 2 parallel, 2 point on line, 1 horizontal, 1 perpendicular
  measures "d108" distance between parallel lines of L7 L5
  measures "d109" distance between parallel lines of L3 L5
extrude "Extrusion6" cut sketch "Sketch6" against normal blind 8 contours L5 L1 L3 L0 | L9 L1 L11 L0
fillet "Fillet4" radius 4 8 edges at (43, -41.5, -17) (18, -41.5, -17) (43, -41.5, -25) (18, -41.5, -25) (-18, -41.5, -17) (-18, -41.5, -25) (-43, -41.5, -17) (-43, -41.5, -25)
sketch "Sketch5" plane through (60, -80, 3) normal (1, 0, 0) x (0, 0, -1)
  line L0 (3, 40) -> (28, 40) projected
  line L1 (15.5, 40) -> (15.5, 0) construction
  line L2 (28, 0) -> (0, 0) projected
  circle A0 centre (15.5, 21) radius 5.5
  point P0 (3, 80)
  dimension "d99" = 11
  dimension "d100" = 19
  constraints: 2 end point, 2 point on line, 1 centre point, 1 midpoint, 1 vertical
  measures "d99" diameter of A0
  measures "d100" distance from line of L0 A0.centre
extrude "Extrusion5" cut sketch "Sketch5" against normal up to surface (3 mm away)
fillet "Fillet1" radius 5 6 edges at (60, 80, 1.5) (60, -80, -11) (-60, -80, -11) (-60, 80, 1.5) (-60, -40, -12.5) (60, -40, -12.5)
fillet "Fillet3" radius 1 8 edges at (48, -43, -12.5) (57, -50, -12.5) (57, -68, -12.5) (48, -77, -12.5) (-48, -77, -12.5) (-57, -68, -12.5) (-57, -50, -12.5) (-48, -43, -12.5)
sketch "Sketch4" plane through (0, 0, 3) normal (0, 0, 1) x (1, 0, 0)
  line L0 (-45, -49) -> (-30, -49)
  line L1 (-30, -49) -> (-30, -70)
  line L2 (-30, -70) -> (-45, -70)
  line L3 (-45, -70) -> (-45, -49)
  line L4 (-60, 75) -> (-60, -75) projected
  line L5 (-55, -80) -> (55, -80) projected
  line L6 (-45, -49) -> (-30, -70) construction
  line L7 (-30, -49) -> (-45, -70) construction
  line L8 (-44, -69) -> (-31, -69)
  line L9 (-31, -69) -> (-31, -50)
  line L10 (-31, -50) -> (-44, -50)
  line L11 (-44, -50) -> (-44, -69)
  line L12 (-44, -69) -> (-31, -50) construction
  line L13 (-31, -69) -> (-44, -50) construction
  point P0 (0, 0)
  point P1 (-37.5, -59.5)
  dimension "d90" = 15
  dimension "d91" = 21
  dimension "d92" = 15
  dimension "d93" = 10
  dimension "d94" = 13
  dimension "d95" = 19
  constraints: 24 end point, 4 parallel, 3 midpoint, 2 horizontal, 2 perpendicular
  measures "d90" distance of L1.end L2.end
  measures "d91" distance of L0.end L1.end
  measures "d92" distance between parallel lines of L4 L3
  measures "d93" distance between parallel lines of L5 L2
  measures "d94" distance of L10.end L9.end
  measures "d95" distance of L9.end L8.end
extrude "Extrusion4" cut sketch "Sketch4" against normal through all contours L11 L10 L9 L8
fillet "Fillet2" radius 0.5 4 edges at (-31, -50, 1.5) (-44, -50, 1.5) (-44, -69, 1.5) (-31, -69, 1.5)
chamfer "Chamfer2" distance 2 angle 45 8 edges at (0, -80, 3) (58.5355, -78.5355, 3) (60, 0, 3) (58.5355, 78.5355, 3) (0, 80, 3) (-58.5355, 78.5355, 3) (-60, 0, 3) (-58.5355, -78.5355, 3)
equation "\"d8\" = d3"
equation "\"d11\" = d2"
equation "\"d66\" = 2 * d63"
body "Solid1"
